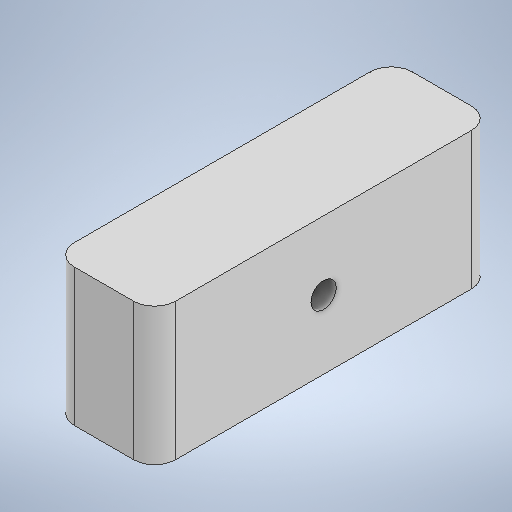
# Autodesk Inventor part: Camera
Saved by Autodesk Inventor 2025.2 (Build 292293000, 293)
## iProperties
Created: 2025-04-06
Part Number: Camera
Material: Generic
Document SubType Name: Modeling
Designer: abdal
Density: 1 g/cm^3
Appearance: Default
Author: abdal
Autodesk Inventor part; units mm, degrees
ref_plane "YZ Plane" through (0, 0, 0) normal (1, 0, 0) x (0, 1, 0)
ref_plane "XZ Plane" through (0, 0, 0) normal (0, 1, 0) x (-1, 0, 0)
sketch "Sketch1" plane through (0, 0, 0) normal (0, 1, 0) x (-1, 0, 0)
  line L0 (12, 40) -> (-12, 40)
  line L1 (-12, 40) -> (-12, -40)
  line L2 (-12, -40) -> (12, -40)
  line L3 (12, -40) -> (12, 40)
  line L4 (12, 40) -> (-12, -40) construction
  line L5 (-12, 40) -> (12, -40) construction
  point P0 (0, 0)
  dimension "d0" = 24
  dimension "d1" = 80
  constraints: 12 end point, 2 midpoint, 2 parallel, 1 horizontal, 1 perpendicular
  measures "d0" distance of L1.end L2.end
  measures "d1" distance of L2.end L0.start
extrude "Extrusion1" add sketch "Sketch1" along normal blind 32.5
sketch "Sketch2" plane through (12, 0, 40) normal (1, 0, 0) x (0, 0, -1)
  circle A0 centre (40, 16.25) radius 3
  line L0 (0, 0) -> (0, 32.5) projected
  line L1 (0, 32.5) -> (80, 32.5) projected
  point P0 (40, 0)
  point P1 (40, 32.5)
  dimension "d4" = 6
  dimension "d5" = 40
  dimension "d6" = 16.25
  constraints: 1 centre point, 1 midpoint
  measures "d4" diameter of A0
  measures "d5" distance from line of L0 A0.centre
  measures "d6" distance of point (40, 32.5) A0.centre
extrude "Extrusion2" cut sketch "Sketch2" against normal blind 5
ref_plane "Work Plane1" through (-12, 0, 0) normal (0, 0, 1) x (1, 0, 0)
sketch "Sketch5" plane through (-12, 0, 0) normal (0, 0, 1) x (1, 0, 0)
  circle A0 centre (-4, 16.25) radius 2
  line L0 (0, 0) -> (0, 32.5) projected
  line L1 (24, 32.5) -> (0, 32.5) projected
  arc A1 (-4, 20.25) -> (-4, 12.25) centre (-4, 16.25) ccw
  line L2 (-4, 12.25) -> (0, 12.25)
  line L3 (-4, 20.25) -> (0, 20.25)
  point P0 (12, 0)
  dimension "d9" = 4
  dimension "d10" = 4
  dimension "d11" = 16.25
  dimension "d12" = 4
  constraints: 4 end point, 2 centre point, 2 perpendicular, 2 point on circle, 2 point on line, 2 tangent, 1 coincident
  measures "d9" diameter of A0
  measures "d10" distance of L2.start A0.centre
  measures "d11" distance from line of L1 A0.centre
  measures "d12" distance from line of L0 A0.centre
extrude "Extrusion3" add sketch "Sketch5" along normal blind 7.5 and the other way blind 7.5
sketch "Sketch7" plane through (-12, 0, -7.5) normal (0, 0, -1) x (-1, 0, 0)
  line L0 (0, 12.25) -> (4, 12.25) projected
  arc A0 (4, 12.25) -> (4, 20.25) centre (4, 16.25) ccw projected
  line L1 (4, 20.25) -> (0, 20.25) projected
  line L2 (0, 12.25) -> (0, 20.25) projected
  circle A1 centre (4, 16.25) radius 2 projected
  line L3 (4, 14.25) -> (7.4641, 14.25)
  line L4 (4, 18.25) -> (7.4641, 18.25)
  point P0 (-12, 0)
  constraints: 4 end point, 4 point on circle, 2 horizontal, 2 tangent
extrude "Extrusion4" cut sketch "Sketch7" against normal blind 2 contours L3 A1 L4 A0
mirror "Mirror1" about plane through (-12, 0, 0) normal (0, 0, 1) of "Extrusion4"
fillet "Fillet2" radius 5 4 edges at (-12, 16.25, 40) (-12, 16.25, -40) (12, 16.25, -40) (12, 16.25, 40)
body "Solid1"
